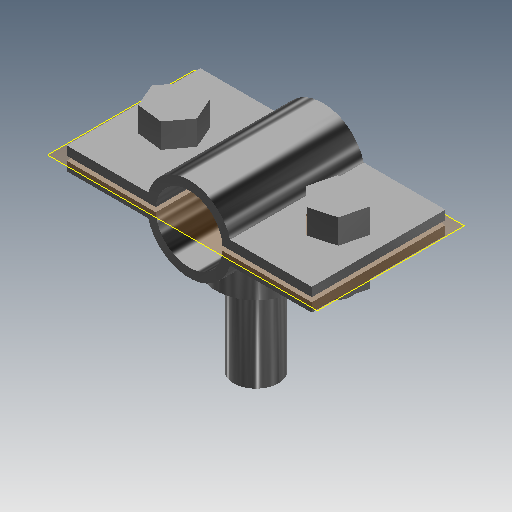
# Autodesk Inventor part: Pipe Clamp - Ø25
Saved by Autodesk Inventor 2020 (Build 240152000, 152)
## iProperties
Created: 2005-11-01
Part Number: Pipe Clamp - Ø25
Document SubType Name: Modeling
Designer: Lars.A.Joergensen
Manufacturer: Standard
Standards Organization: Custom
Description: Pipe Support
Density: 8 g/cm^3
Material: Stainless Steel
Mass: 102.407 g
Surface Area: 99.8895 cm^2
Volume: 12.8009 cm^3
Stock Number: NA
Appearance: Chrome - Polished Black
Title: Purchased Part
Author: Demir Ali
Revision Number: A
Autodesk Inventor part; units mm, degrees
sketch "Sketch1" plane through (0, 0, 0) normal (0, 0, 1) x (1, 0, 0)
  circle A0 centre (0, 0) radius 7.5
  circle A1 centre (0, 0) radius 9.5
  dimension "d0" = 15
  dimension "d1" = 2
  constraints: 2 centre point, 2 coincident
  measures "d0" diameter of A0
  measures "d1" radial gap between concentric circles of A0 A1
extrude "Extrusion1" add sketch "Sketch1" along normal mid plane 30
sketch "Sketch3" plane through (0, 0, 0) normal (0, 0, 1) x (1, 0, 0)
  circle A0 centre (0, 0) radius 9.5 projected
  line L0 (-27.5, 2.5) -> (-27.5, -2.5)
  line L1 (-27.5, 2.5) -> (-9.1652, 2.5)
  line L2 (-27.5, -2.5) -> (-9.1652, -2.5)
  line L3 (27.5, 2.5) -> (27.5, -2.5)
  line L4 (27.5, 2.5) -> (9.1652, 2.5)
  line L5 (27.5, -2.5) -> (9.1652, -2.5)
  point P0 (-27.5, 0)
  point P1 (27.5, 0)
  dimension "d4" = 5
  dimension "d6" = 5
  dimension "d22" = 27.5
  dimension "d23" = 27.5
  constraints: 12 end point, 4 point on circle, 3 perpendicular, 2 horizontal alignment, 2 midpoint, 2 parallel, 1 vertical
  measures "d4" distance of L0.start L0.end
  measures "d6" distance of L3.start L3.end
  measures "d22" distance of point (-27.5, 0) A0.centre
  measures "d23" distance of point (27.5, 0) A0.centre
extrude "Extrusion2" add sketch "Sketch3" along normal mid plane 30 contours A0 L4 L3 L5 | A0 L2 L0 L1
sketch "Sketch10" plane through (0, 0, 0) normal (0, 0, 1) x (1, 0, 0)
  line L0 (-27.5, -2.5) -> (-27.5, 2.5) projected
  line L1 (27.5, 2.5) -> (27.5, -2.5) projected
  line L2 (-27.5, -0.5) -> (27.5, -0.5)
  line L3 (27.5, -0.5) -> (27.5, 0.5)
  line L4 (27.5, 0.5) -> (-27.5, 0.5)
  line L5 (-27.5, 0.5) -> (-27.5, -0.5)
  line L6 (27.5, -2.5) -> (9.1652, -2.5) projected
  line L7 (9.1652, 2.5) -> (27.5, 2.5) projected
  point P0 (0, 0)
  dimension "d28" = 2
  dimension "d29" = 2
  constraints: 8 end point, 2 parallel, 2 point on line, 1 horizontal, 1 perpendicular
  measures "d28" distance between parallel lines of L6 L2
  measures "d29" distance between parallel lines of L7 L4
extrude "Extrusion7" cut sketch "Sketch10" along normal through all both and the other way through all
sketch "Sketch4" plane through (-27.5, -2.5, -15) normal (0, -1, 0) x (1, 0, 0)
  line L0 (18.3348, 30) -> (0, 30) projected
  line L1 (0, 0) -> (0, 30) projected
  line L2 (55, 30) -> (36.6652, 30) projected
  line L3 (36.6652, 0) -> (36.6652, 30) projected
  line L4 (36.6652, 0) -> (55, 0) projected
  line L5 (55, 0) -> (55, 30) projected
  circle A0 centre (9.1674, 15) radius 3
  circle A1 centre (45.8326, 15) radius 3
  point P0 (0, 15)
  point P1 (9.1674, 30)
  point P2 (45.8326, 30)
  point P3 (55, 15)
  dimension "d10" = 6
  dimension "d11" = 6
  constraints: 4 midpoint, 2 centre point, 2 horizontal alignment, 2 vertical alignment
  measures "d10" diameter of A0
  measures "d11" diameter of A1
extrude "Extrusion3" add sketch "Sketch4" along normal mid plane 15 contours A0 | A1
ref_plane "Work Plane1" through (0, 8, 0) normal (0, 1, 0) x (-1, 0, 0)
sketch "Sketch6" plane through (0, 8, 0) normal (0, 1, 0) x (-1, 0, 0)
  circle A0 centre (-18.3326, 0) radius 3 projected
  circle A1 centre (18.3326, 0) radius 3 projected
  line L0 (-19.7333, -5.601) -> (-23.8836, -1.5874)
  line L1 (-23.8836, -1.5874) -> (-22.4828, 4.0136)
  line L2 (-22.4828, 4.0136) -> (-16.9318, 5.601)
  line L3 (-16.9318, 5.601) -> (-12.7816, 1.5874)
  line L4 (-12.7816, 1.5874) -> (-14.1824, -4.0136)
  line L5 (-14.1824, -4.0136) -> (-19.7333, -5.601)
  line L6 (20.6316, -5.296) -> (14.8956, -4.639)
  line L7 (14.8956, -4.639) -> (12.5966, 0.657)
  line L8 (12.5966, 0.657) -> (16.0335, 5.296)
  line L9 (16.0335, 5.296) -> (21.7695, 4.639)
  line L10 (21.7695, 4.639) -> (24.0686, -0.657)
  line L11 (24.0686, -0.657) -> (20.6316, -5.296)
  dimension "d15" = 10
  constraints: 24 end point, 2 coincident, 1 equal length, 22 other
  measures "d15" distance between parallel lines of L2 L5
extrude "Extrusion4" add sketch "Sketch6" against normal up to surface (5.5 mm away) contours A0 | A1 | L0 L1 L2 L3 L4 L5 | L6 L7 L8 L9 L10 L11
ref_plane "Length_WKP" through (0, -35, 0) normal (0, 1, 0) x (-1, 0, 0)
sketch "Sketch8" plane through (0, -35, 0) normal (0, 1, 0) x (-1, 0, 0)
  line L0 (-38.5, 0) -> (38.5, 0) projected
  line L1 (0, -21) -> (0, 21) projected
  circle A0 centre (0, 0) radius 5
  dimension "d19" = 10
  constraints: 2 midpoint, 1 centre point
  measures "d19" diameter of A0
extrude "Extrusion5" add sketch "Sketch8" along normal up to next
ref_plane "Work Plane3" through (0, -15, 0) normal (0, 1, 0) x (-1, 0, 0)
sketch "Sketch9" plane through (0, -15, 0) normal (0, 1, 0) x (-1, 0, 0)
  circle A0 centre (0, 0) radius 5 projected
  circle A1 centre (0, 0) radius 9
  dimension "d25" = 4
  constraints: 1 centre point
  measures "d25" radial gap between concentric circles of A1 A0
extrude "Extrusion6" add sketch "Sketch9" along normal up to next
mirror "Mirror1" about plane through (0, 0, 0) normal (0, 1, 0) of "Extrusion4"
equation "\"d0\" = dia"
equation "\"d2\" = Bredde"
equation "\"d8\" = Bredde"
equation "\"d29\" = d28"
equation "\"d11\" = d10"
equation "\"dia\" = 15"
equation "\"Bredde\" = 30"
body "Solid1"
